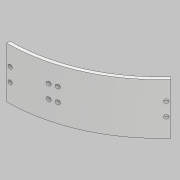
# Autodesk Inventor part: CW004
Saved by Autodesk Inventor 2017 (Build 210142000, 142)
## iProperties
Created: 2017-05-24
Part Number: CW004
Material: ABS Plastic
Document SubType Name: Modeling
Designer: zallen
Density: 1.06 g/cm^3
Appearance: CR White
Author: zallen
Autodesk Inventor part; units mm, degrees
ref_plane "YZ Plane" through (0, 0, 0) normal (1, 0, 0) x (0, 1, 0)
sketch "Sketch1" plane through (0, 0, 0) normal (0, 0, 1) x (1, 0, 0)
  circle A0 centre (0, 225) radius 225 construction
  circle A1 centre (0, 225) radius 220 construction
  line L0 (0, 5) -> (0, 0)
  arc A2 (0, 0) -> (167.5, 74.771) centre (0, 225) ccw
  line L1 (167.5, 74.771) -> (163.7778, 78.1094)
  arc A3 (0, 5) -> (163.7778, 78.1094) centre (0, 225) ccw
  dimension "d0" = 450
  dimension "d1" = 5
  dimension "d2" = 5
  dimension "d3" = 167.5
  constraints: 8 point on circle, 4 centre point, 4 end point, 3 concentric, 1 vertical, 1 vertical alignment
  measures "d0" diameter of A0
  measures "d1" radial gap between concentric circles of A0 A1
  measures "d2" distance of L1.start L1.end
  measures "d3" horizontal distance of L1.start L0.end
extrude "Extrusion1" add sketch "Sketch1" along normal blind 75
ref_plane "Work Plane1" through (167.5, 74.771, 0) normal (0.7444, -0.6677, 0) x (0.6677, 0.7444, 0)
sketch "Sketch2" plane through (167.5, 74.771, 0) normal (0.7444, -0.6677, 0) x (0.6677, 0.7444, 0)
  circle A0 centre (-5, 47.5) radius 3
  circle A1 centre (-5, 27.5) radius 3
  line L0 (0, 0) -> (-167.5, 0) projected
  line L1 (0, 0) -> (0, 75) projected
  line L2 (-167.5, 75) -> (0, 75) projected
  line L3 (-167.5, 0) -> (-167.5, 75) projected
  dimension "d6" = 6
  dimension "d7" = 6
  dimension "d8" = 5
  dimension "d9" = 27.5
  dimension "d10" = 20
  constraints: 2 centre point, 1 vertical alignment
  measures "d6" diameter of A0
  measures "d7" diameter of A1
  measures "d8" horizontal distance of L0.start A1.centre
  measures "d9" vertical distance of L0.start A1.centre
  measures "d10" distance of A1.centre A0.centre
extrude "Extrusion2" cut sketch "Sketch2" along normal through all both and the other way through all contours A0 | A1
ref_plane "Work Plane2" through (0, 0, 0) normal (0, -1, 0) x (1, 0, 0)
sketch "Sketch3" plane through (0, 0, 0) normal (0, -1, 0) x (1, 0, 0)
  circle A0 centre (5, 47.5) radius 3
  circle A1 centre (5, 27.5) radius 3
  circle A2 centre (55, 47.5) radius 3
  circle A3 centre (55, 27.5) radius 3
  circle A4 centre (65.5, 47.5) radius 3
  circle A5 centre (65.5, 27.5) radius 3
  point P0 (0, 0)
  dimension "d13" = 6
  dimension "d14" = 6
  dimension "d15" = 6
  dimension "d16" = 6
  dimension "d17" = 27.5
  dimension "d18" = 20
  dimension "d19" = 5
  dimension "d20" = 55
  dimension "d23" = 6
  dimension "d24" = 6
  dimension "d25" = 10.5
  constraints: 6 centre point, 4 horizontal alignment, 3 vertical alignment
  measures "d13" diameter of A0
  measures "d14" diameter of A1
  measures "d15" diameter of A2
  measures "d16" diameter of A3
  measures "d17" vertical distance of point (0, 0) A1.centre
  measures "d18" distance of A0.centre A1.centre
  measures "d19" horizontal distance of point (0, 0) A1.centre
  measures "d20" horizontal distance of A3.centre point (0, 0)
  measures "d23" diameter of A4
  measures "d24" diameter of A5
  measures "d25" distance of A5.centre A3.centre
extrude "Extrusion3" cut sketch "Sketch3" along normal through all both and the other way through all
body "Solid1"
